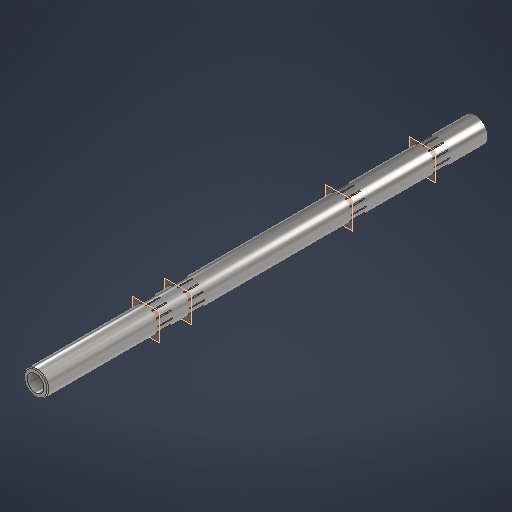
# Autodesk Inventor part: Albero Cavo
Saved by Autodesk Inventor 2026.2 (Build 302298010, 298A)
## iProperties
Created: 2026-04-14
Part Number: Albero Cavo
Material: Stainless Steel
Document SubType Name: Modeling
Designer: Yan
Density: 8 g/cm^3
Appearance: Semi-Polished
Author: Yan
Autodesk Inventor part; units mm, degrees
note: some values were not read from the file. Chosen so that the rebuilt part matches the saved one: pattern direction of "Circular Pattern1"; pattern direction of "Circular Pattern2"; pattern direction of "Circular Pattern3"; pattern direction of "Circular Pattern4".
ref_plane "YZ Plane" through (0, 0, 0) normal (1, 0, 0) x (0, 1, 0)
ref_plane "XZ Plane" through (0, 0, 0) normal (0, 1, 0) x (-1, 0, 0)
ref_plane "XY Plane" through (0, 0, 0) normal (0, 0, 1) x (1, 0, 0)
sketch "Sketch1" plane through (0, 0, 0) normal (1, 0, 0) x (0, 1, 0)
  line L0 (0, 0) -> (0, -1800)
  line L1 (0, -1800) -> (50, -1800)
  line L2 (50, -1800) -> (50, 0)
  line L3 (50, 0) -> (0, 0)
  dimension "d22" = 1800
  dimension "d23" = 100
  constraints: 8 end point, 3 perpendicular, 1 vertical
  measures "d22" distance between parallel lines of L1 L3
  measures "d23" diameter of L2 L0
revolve "Revolution1" add sketch "Sketch1" angle 360 about axis through (0, 0, 0) along (0, 0, -1)
sketch "Sketch2" plane through (0, 0, 0) normal (0, 0, 1) x (1, 0, 0)
  point P0 (0, 0)
  point P1 (0, 0)
  constraints: 1 coincident
hole "Hole1" at (0, 0, 0) direction (0, 0, -1) diameter 68 end through all
ref_plane "Work Plane1" through (0, 0, -450) normal (0, 0, 1) x (1, 0, 0)
sketch "Sketch3" plane through (0, 0, -450) normal (0, 0, 1) x (1, 0, 0)
  line L0 (-2, 47.5) -> (2, 47.5)
  line L1 (2, 47.5) -> (2, 52.5)
  line L2 (2, 52.5) -> (-2, 52.5)
  line L3 (-2, 52.5) -> (-2, 47.5)
  circle A0 centre (0, 0) radius 50 projected
  line L4 (-2, 47.5) -> (2, 52.5) construction
  line L5 (2, 47.5) -> (-2, 52.5) construction
  point P0 (0, 50)
  point P1 (2, 49.96)
  point P2 (-2, 49.96)
  dimension "d34" = 4
  dimension "d35" = 52.5
  dimension "d36" = 0
  constraints: 12 end point, 2 midpoint, 2 parallel, 1 horizontal, 1 perpendicular, 2 other
  measures "d34" distance between parallel lines of L1 L3
  measures "d35" distance from line of point (0, 0) L2
  measures "d36" horizontal distance of point (0, 0) point (0, 50)
extrude "Extrusion1" cut sketch "Sketch3" against normal blind 60 contours L3 A0 L1 L0 picked at (-0.2223, 48.3319)
chamfer "Chamfer1" distance 4 angle 30 1 edges at (0, 47.5, -450) measured on face at (-0.6667, 47.5, -470)
chamfer "Chamfer2" distance 4 angle 30 1 edges at (0, 47.5, -510) measured on face at (-0.6667, 47.5, -491.3333)
pattern_circular "Circular Pattern1" count 12 over 360 about axis through (0, 0, -10) along (0, 0, 1) of "Extrusion1"
ref_plane "Work Plane2" through (0, 0, -580) normal (0, 0, 1) x (1, 0, 0)
sketch "Sketch4" plane through (0, 0, -580) normal (0, 0, 1) x (1, 0, 0)
  line L0 (-52.5, -2) -> (-47.5, -2)
  line L1 (-47.5, -2) -> (-47.5, 2)
  line L2 (-47.5, 2) -> (-52.5, 2)
  line L3 (-52.5, 2) -> (-52.5, -2)
  line L4 (-52.5, -2) -> (-47.5, 2) construction
  line L5 (-47.5, -2) -> (-52.5, 2) construction
  circle A0 centre (0, 0) radius 50 projected
  point P0 (-50, 0)
  point P1 (-49.96, 2)
  point P2 (-49.96, -2)
  dimension "d49" = 4
  dimension "d50" = 50
  dimension "d51" = 0
  dimension "d52" = 47.5
  constraints: 12 end point, 2 midpoint, 2 parallel, 1 horizontal, 1 perpendicular
  measures "d49" distance between parallel lines of L2 L0
  measures "d50" distance of point (0, 0) point (-50, 0)
  measures "d51" vertical distance of A0.centre point (-50, 0)
  measures "d52" distance from line of point (0, 0) L1
extrude "Extrusion2" cut sketch "Sketch4" against normal blind 60 contours A0 L2 L1 L0 picked at (-48.3319, -0.2223)
chamfer "Chamfer3" distance 4 angle 30 2 edges at (-47.5, 0, -640) (-47.5, 0, -580) measured on face at (-47.5, -0.6667, -600)
pattern_circular "Circular Pattern2" count 12 over 360 about axis through (0, 0, -10) along (0, 0, 1) of "Extrusion2"
ref_plane "Work Plane3" through (0, 0, -1240) normal (0, 0, 1) x (1, 0, 0)
sketch "Sketch5" plane through (0, 0, -1240) normal (0, 0, 1) x (1, 0, 0)
  line L0 (-47.5, -2) -> (-52.5, -2)
  line L1 (-52.5, -2) -> (-52.5, 2)
  line L2 (-52.5, 2) -> (-47.5, 2)
  line L3 (-47.5, 2) -> (-47.5, -2)
  line L4 (-47.5, -2) -> (-52.5, 2) construction
  line L5 (-52.5, -2) -> (-47.5, 2) construction
  circle A0 centre (0, 0) radius 50 projected
  point P0 (-50, 0)
  point P1 (-49.96, 2)
  point P2 (-49.96, -2)
  dimension "d62" = 4
  dimension "d64" = 47.5
  dimension "d65" = 50
  dimension "d66" = 5
  constraints: 12 end point, 2 midpoint, 2 parallel, 1 horizontal, 1 perpendicular
  measures "d62" distance between parallel lines of L2 L0
  measures "d64" distance from line of point (0, 0) L3
  measures "d65" distance of A0.centre point (-50, 0)
  measures "d66" distance of L1.end L2.end
extrude "Extrusion3" cut sketch "Sketch5" against normal blind 60 contours L0 A0 L2 L3 picked at (-48.3319, -0.2223)
chamfer "Chamfer4" distance 4 angle 30 2 edges at (-47.5, 0, -1300) (-47.5, 0, -1240) measured on face at (-47.5, -0.6667, -1260)
pattern_circular "Circular Pattern3" count 12 over 360 about axis through (0, 0, -10) along (0, 0, 1) of "Extrusion3"
ref_plane "Work Plane4" through (0, 0, -1580) normal (0, 0, 1) x (1, 0, 0)
sketch "Sketch6" plane through (0, 0, -1580) normal (0, 0, 1) x (1, 0, 0)
  line L0 (-47.5, 2) -> (-52.5, 2)
  line L1 (-52.5, 2) -> (-52.5, -2)
  line L2 (-52.5, -2) -> (-47.5, -2)
  line L3 (-47.5, -2) -> (-47.5, 2)
  line L4 (-47.5, 2) -> (-52.5, -2) construction
  line L5 (-52.5, 2) -> (-47.5, -2) construction
  circle A0 centre (0, 0) radius 50 projected
  point P0 (-50, 0)
  point P1 (-49.96, 2)
  point P2 (-49.96, -2)
  dimension "d76" = 4
  dimension "d77" = 5
  dimension "d78" = 47.5
  dimension "d79" = 0
  constraints: 12 end point, 2 midpoint, 2 parallel, 1 horizontal, 1 perpendicular
  measures "d76" distance between parallel lines of L0 L2
  measures "d77" distance between parallel lines of L3 L1
  measures "d78" distance from line of point (0, 0) L3
  measures "d79" vertical distance of A0.centre point (-50, 0)
extrude "Extrusion4" cut sketch "Sketch6" against normal blind 60 contours L3 L2 A0 L0 picked at (-48.3319, -0.2223)
chamfer "Chamfer5" distance 4 angle 30 2 edges at (-47.5, 0, -1640) (-47.5, 0, -1580) measured on face at (-47.5, -0.6667, -1600)
pattern_circular "Circular Pattern4" count 12 over 360 about axis through (0, 0, -10) along (0, 0, 1) of "Extrusion4"
chamfer "Chamfer6" distance 4 angle 45 2 edges at (0, -50, 0) (0, -50, -1800)
chamfer "Chamfer7" distance 4 angle 30 2 edges at (-47.5, 0, -450) (-47.5, 0, -510) measured on face at (-47.5, -0.6667, -470)
chamfer "Chamfer8" distance 4 angle 30 2 edges at (-41.1362, 23.75, -510) (-41.1362, 23.75, -450) measured on face at (-41.4695, 23.1726, -470)
chamfer "Chamfer9" distance 4 angle 30 2 edges at (-23.75, 41.1362, -450) (-23.75, 41.1362, -510) measured on face at (-24.3274, 40.8029, -470)
chamfer "Chamfer10" distance 4 angle 30 2 edges at (23.75, 41.1362, -510) (23.75, 41.1362, -450) measured on face at (23.1726, 41.4695, -470)
chamfer "Chamfer11" distance 4 angle 30 2 edges at (41.1362, 23.75, -510) (41.1362, 23.75, -450) measured on face at (40.8029, 24.3274, -470)
chamfer "Chamfer12" distance 4 angle 30 2 edges at (47.5, 0, -510) (47.5, 0, -450) measured on face at (47.5, 0.6667, -470)
chamfer "Chamfer13" distance 4 angle 30 2 edges at (41.1362, -23.75, -510) (41.1362, -23.75, -450) measured on face at (41.4695, -23.1726, -470)
chamfer "Chamfer14" distance 4 angle 30 2 edges at (23.75, -41.1362, -510) (23.75, -41.1362, -450) measured on face at (24.3274, -40.8029, -470)
chamfer "Chamfer15" distance 4 angle 30 2 edges at (0, -47.5, -510) (0, -47.5, -450) measured on face at (0.6667, -47.5, -470)
chamfer "Chamfer16" distance 4 angle 30 2 edges at (-23.75, -41.1362, -510) (-23.75, -41.1362, -450) measured on face at (-23.1726, -41.4695, -470)
chamfer "Chamfer17" distance 4 angle 30 2 edges at (-41.1362, -23.75, -510) (-41.1362, -23.75, -450) measured on face at (-40.8029, -24.3274, -470)
chamfer "Chamfer18" distance 4 angle 30 2 edges at (-23.75, 41.1362, -580) (-23.75, 41.1362, -640) measured on face at (-24.3274, 40.8029, -600)
chamfer "Chamfer19" distance 4 angle 30 2 edges at (-41.1362, 23.75, -640) (-41.1362, 23.75, -580) measured on face at (-41.4695, 23.1726, -600)
chamfer "Chamfer20" distance 4 angle 30 2 edges at (-41.1362, -23.75, -580) (-41.1362, -23.75, -640) measured on face at (-40.8029, -24.3274, -600)
chamfer "Chamfer21" distance 4 angle 30 2 edges at (-23.75, -41.1362, -640) (-23.75, -41.1362, -580) measured on face at (-23.1726, -41.4695, -600)
chamfer "Chamfer22" distance 4 angle 30 2 edges at (0, -47.5, -640) (0, -47.5, -580) measured on face at (0.6667, -47.5, -600)
chamfer "Chamfer23" distance 4 angle 30 2 edges at (23.75, -41.1362, -640) (23.75, -41.1362, -580) measured on face at (24.3274, -40.8029, -600)
chamfer "Chamfer24" distance 4 angle 30 2 edges at (41.1362, -23.75, -640) (41.1362, -23.75, -580) measured on face at (41.4695, -23.1726, -600)
chamfer "Chamfer25" distance 4 angle 30 2 edges at (47.5, 0, -640) (47.5, 0, -580) measured on face at (47.5, 0.6667, -600)
chamfer "Chamfer26" distance 4 angle 30 2 edges at (41.1362, 23.75, -640) (41.1362, 23.75, -580) measured on face at (40.8029, 24.3274, -600)
chamfer "Chamfer27" distance 4 angle 30 2 edges at (23.75, 41.1362, -640) (23.75, 41.1362, -580) measured on face at (23.1726, 41.4695, -600)
chamfer "Chamfer28" distance 4 angle 30 2 edges at (0, 47.5, -640) (0, 47.5, -580) measured on face at (-0.6667, 47.5, -600)
chamfer "Chamfer29" distance 4 angle 30 2 edges at (0, 47.5, -1300) (0, 47.5, -1240) measured on face at (-0.6667, 47.5, -1260)
chamfer "Chamfer30" distance 4 angle 30 2 edges at (-23.75, 41.1362, -1300) (-23.75, 41.1362, -1240) measured on face at (-24.3274, 40.8029, -1260)
chamfer "Chamfer31" distance 4 angle 30 2 edges at (-41.1362, 23.75, -1300) (-41.1362, 23.75, -1240) measured on face at (-41.4695, 23.1726, -1260)
chamfer "Chamfer32" distance 4 angle 30 2 edges at (-41.1362, -23.75, -1300) (-41.1362, -23.75, -1240) measured on face at (-40.8029, -24.3274, -1260)
chamfer "Chamfer33" distance 4 angle 30 2 edges at (-23.75, -41.1362, -1300) (-23.75, -41.1362, -1240) measured on face at (-23.1726, -41.4695, -1260)
chamfer "Chamfer34" distance 4 angle 30 2 edges at (0, -47.5, -1300) (0, -47.5, -1240) measured on face at (0.6667, -47.5, -1260)
chamfer "Chamfer35" distance 4 angle 30 2 edges at (23.75, -41.1362, -1300) (23.75, -41.1362, -1240) measured on face at (24.3274, -40.8029, -1260)
chamfer "Chamfer36" distance 4 angle 30 2 edges at (41.1362, -23.75, -1300) (41.1362, -23.75, -1240) measured on face at (41.4695, -23.1726, -1260)
chamfer "Chamfer37" distance 4 angle 30 2 edges at (47.5, 0, -1300) (47.5, 0, -1240) measured on face at (47.5, 0.6667, -1260)
chamfer "Chamfer38" distance 4 angle 30 2 edges at (41.1362, 23.75, -1300) (41.1362, 23.75, -1240) measured on face at (40.8029, 24.3274, -1260)
chamfer "Chamfer39" distance 4 angle 30 2 edges at (23.75, 41.1362, -1300) (23.75, 41.1362, -1240) measured on face at (23.1726, 41.4695, -1260)
chamfer "Chamfer40" distance 4 angle 30 2 edges at (0, 47.5, -1640) (0, 47.5, -1580) measured on face at (-0.6667, 47.5, -1600)
chamfer "Chamfer41" distance 4 angle 30 2 edges at (-23.75, 41.1362, -1640) (-23.75, 41.1362, -1580) measured on face at (-24.3274, 40.8029, -1600)
chamfer "Chamfer42" distance 4 angle 30 2 edges at (-41.1362, 23.75, -1580) (-41.1362, 23.75, -1640) measured on face at (-41.4695, 23.1726, -1600)
chamfer "Chamfer43" distance 4 angle 30 2 edges at (-41.1362, -23.75, -1640) (-41.1362, -23.75, -1580) measured on face at (-40.8029, -24.3274, -1600)
chamfer "Chamfer44" distance 4 angle 30 2 edges at (-23.75, -41.1362, -1640) (-23.75, -41.1362, -1580) measured on face at (-23.1726, -41.4695, -1600)
chamfer "Chamfer45" distance 4 angle 30 2 edges at (0, -47.5, -1640) (0, -47.5, -1580) measured on face at (0.6667, -47.5, -1600)
chamfer "Chamfer46" distance 4 angle 30 2 edges at (23.75, -41.1362, -1640) (23.75, -41.1362, -1580) measured on face at (24.3274, -40.8029, -1600)
chamfer "Chamfer47" distance 4 angle 30 2 edges at (41.1362, -23.75, -1640) (41.1362, -23.75, -1580) measured on face at (41.4695, -23.1726, -1600)
chamfer "Chamfer48" distance 4 angle 30 2 edges at (47.5, 0, -1640) (47.5, 0, -1580) measured on face at (47.5, 0.6667, -1600)
chamfer "Chamfer49" distance 4 angle 30 2 edges at (41.1362, 23.75, -1640) (41.1362, 23.75, -1580) measured on face at (40.8029, 24.3274, -1600)
chamfer "Chamfer50" distance 4 angle 30 2 edges at (23.75, 41.1362, -1640) (23.75, 41.1362, -1580) measured on face at (23.1726, 41.4695, -1600)
body "Solid1"
